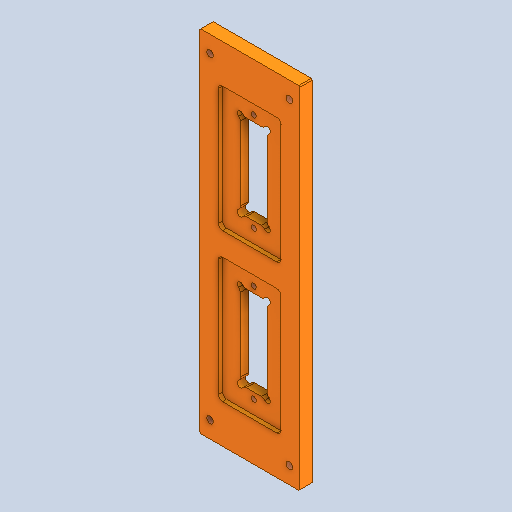
# Autodesk Inventor part: Regua DB25-berço
Saved by Autodesk Inventor 2026 (Build 300175050, 175E)
## iProperties
Created: 2025-09-19
Part Number: Regua DB25-berço
Material: Fenolite OR
Document SubType Name: Modeling
Designer: Kedson Neves
Density: 1.4 g/cm^3
Appearance: Genérico(1)
Author: Kedson Neves
Autodesk Inventor part; units mm, degrees
ref_plane "YZ Plane" through (0, 0, 0) normal (1, 0, 0) x (0, 1, 0)
ref_plane "XZ Plane" through (0, 0, 0) normal (0, 1, 0) x (-1, 0, 0)
ref_plane "XY Plane" through (0, 0, 0) normal (0, 0, 1) x (1, 0, 0)
sketch "Esboço1" plane through (0, 0, 0) normal (0, 0, 1) x (1, 0, 0)
  line L0 (24.0444, 83.9778) -> (-23.9556, 83.9778)
  line L1 (-23.9556, 83.9778) -> (-23.9556, -84.0222)
  line L2 (-23.9556, -84.0222) -> (24.0444, -84.0222)
  line L3 (24.0444, -84.0222) -> (24.0444, 83.9778)
  circle A0 centre (19.0444, 75.9778) radius 2.25
  circle A1 centre (-18.9556, 75.9778) radius 2.25
  circle A2 centre (-18.9556, -76.0222) radius 2.25
  circle A3 centre (19.0444, -76.0222) radius 2.25
  point P0 (0, 0)
  dimension "d0" = 5
  dimension "d1" = 5
  dimension "d2" = 8
  dimension "d3" = 8
  constraints: 8 end point, 4 centre point, 2 parallel, 1 horizontal, 1 perpendicular
  measures "d0" distance from line of A0.centre L3
  measures "d1" distance from line of A1.centre L1
  measures "d2" distance from line of A1.centre L0
  measures "d3" distance from line of L2 A2.centre
extrude "Extrusão1" add sketch "Esboço1" along normal blind 6
sketch "Esboço2" plane through (0, 0, 6) normal (0, 0, 1) x (1, 0, 0)
  line L0 (-10.5, 71) -> (10.5, 71)
  line L1 (10.5, 71) -> (10.5, -71)
  line L2 (10.5, -71) -> (-10.5, -71)
  line L3 (-10.5, -71) -> (-10.5, 71)
  line L4 (-10.5, 71) -> (10.5, -71) construction
  line L5 (10.5, 71) -> (-10.5, -71) construction
  line L6 (10.5, 71) -> (-10.5, 0)
  line L7 (-6.5, 56) -> (6.5, 56)
  line L8 (6.5, 56) -> (6.5, 15)
  line L9 (6.5, 15) -> (-6.5, 15)
  line L10 (-6.5, 15) -> (-6.5, 56)
  line L11 (-6.5, 56) -> (6.5, 15) construction
  line L12 (6.5, 56) -> (-6.5, 15) construction
  circle A0 centre (-6.5, 56) radius 1.5
  circle A1 centre (-6.5, 15) radius 1.5
  circle A2 centre (6.5, 15) radius 1.5
  circle A3 centre (6.5, 56) radius 1.5
  line L13 (10.5, 0) -> (-10.5, 0)
  line L14 (-6.5, -56) -> (6.5, -56)
  line L15 (6.5, -56) -> (6.5, -15)
  line L16 (6.5, -15) -> (-6.5, -15)
  line L17 (-6.5, -15) -> (-6.5, -56)
  circle A4 centre (-6.5, -56) radius 1.5
  circle A5 centre (-6.5, -15) radius 1.5
  circle A6 centre (6.5, -15) radius 1.5
  circle A7 centre (6.5, -56) radius 1.5
  point P0 (0, 0)
  point P1 (0, 35.5)
  point P2 (5, -15)
  point P3 (-5, -15)
  point P4 (-6.5, -16.5)
  point P5 (-6.5, -54.5)
  point P6 (-5, -56)
  point P7 (5, -56)
  point P8 (6.5, -54.5)
  point P9 (6.5, -16.5)
  point P10 (-5, 15)
  point P11 (5, 15)
  point P12 (6.5, 16.5)
  point P13 (6.5, 54.5)
  point P14 (5, 56)
  point P15 (-5, 56)
  point P16 (-6.5, 54.5)
  point P17 (-6.5, 16.5)
  dimension "d6" = 142
  dimension "d7" = 21
  dimension "d8" = 41
  dimension "d9" = 13
  dimension "d10" = 3
  constraints: 36 end point, 8 centre point, 8 coincident, 8 symmetric about line, 7 midpoint, 5 equal radius, 4 parallel, 3 perpendicular, 2 horizontal, 4 other
  measures "d6" distance of L0.end L1.end
  measures "d7" distance of L0.start L0.end
  measures "d8" distance of L7.end L8.end
  measures "d9" distance of L7.start L7.end
  measures "d10" diameter of A3
extrude "Extrusão2" cut sketch "Esboço2" against normal through all contours A3 L8 L7 L6 | L6 L7 A3 | A1 L10 L9 L6 | L6 L9 A1 | L7 L8 A3 L6 | L6 A3 L7 | A3 L6 A1 L10 A0 L7 | L9 L10 A1 L6 | L6 A1 L9 | A1 L6 A3 L8 A2 L9 | A0 L10 L7 | L7 L10 A0 | A2 L8 L9 | L9 L8 A2 | L17 A4 L14 | L14 A4 L17 | A4 L17 A5 L16 A6 L15 A7 L14 | A7 L15 L14 | L14 L15 A7 | A5 L16 L17 | L17 L16 A5 | A6 L16 L15 | L15 L16 A6
fillet "Arredondamento1" radius 2 16 edges at (6.5, 16.5, 3) (5, 15, 3) (-5, 15, 3) (-6.5, 16.5, 3) (-6.5, 54.5, 3) (-5, 56, 3) (5, 56, 3) (6.5, 54.5, 3) (6.5, -16.5, 3) (5, -15, 3) (-6.5, -16.5, 3) (-5, -15, 3) (-6.5, -54.5, 3) (-5, -56, 3) (5, -56, 3) (6.5, -54.5, 3)
sketch "Esboço3" plane through (0, 0, 6) normal (0, 0, 1) x (1, 0, 0)
  line L0 (6.5, 53.1277) -> (6.5, 17.8723) projected
  line L1 (6.5, 35.5) -> (-6.5, 35.5)
  line L2 (-6.5, 17.8723) -> (-6.5, 53.1277) projected
  line L3 (6.5, -53.1277) -> (6.5, -17.8723) projected
  line L4 (6.5, -35.5) -> (-6.5, -35.5)
  line L5 (-6.5, -17.8723) -> (-6.5, -53.1277) projected
  line L6 (-15, 65.5) -> (15, 65.5)
  line L7 (15, 65.5) -> (15, 5.5)
  line L8 (15, 5.5) -> (-15, 5.5)
  line L9 (-15, 5.5) -> (-15, 65.5)
  line L10 (-15, 65.5) -> (15, 5.5) construction
  line L11 (15, 65.5) -> (-15, 5.5) construction
  line L12 (-15, -5.5) -> (15, -5.5)
  line L13 (15, -5.5) -> (15, -65.5)
  line L14 (15, -65.5) -> (-15, -65.5)
  line L15 (-15, -65.5) -> (-15, -5.5)
  line L16 (-15, -5.5) -> (15, -65.5) construction
  line L17 (15, -5.5) -> (-15, -65.5) construction
  point P0 (0, 0)
  point P1 (0, 35.5)
  point P2 (0, -35.5)
  dimension "d14" = 60
  dimension "d15" = 30
  dimension "d16" = 60
  dimension "d17" = 30
  constraints: 28 end point, 10 midpoint, 4 parallel, 2 horizontal, 2 perpendicular
  measures "d14" distance of L6.end L7.end
  measures "d15" distance of L6.start L6.end
  measures "d16" distance of L12.end L13.end
  measures "d17" distance of L12.start L12.end
extrude "Extrusão3" cut sketch "Esboço3" against normal blind 2
fillet "Arredondamento2" radius 2 8 edges at (15, 65.5, 5) (-15, 65.5, 5) (-15, 5.5, 5) (15, 5.5, 5) (15, -5.5, 5) (-15, -5.5, 5) (-15, -65.5, 5) (15, -65.5, 5)
sketch "Esboço4" plane through (0, 0, 4) normal (0, 0, 1) x (1, 0, 0)
  line L0 (6.5, 17.8723) -> (6.5, 53.1277) projected
  line L1 (6.5, 35.5) -> (-6.5, 35.5)
  line L2 (-6.5, 53.1277) -> (-6.5, 17.8723) projected
  line L3 (6.5, -53.1277) -> (6.5, -17.8723) projected
  line L4 (6.5, -35.5) -> (-6.5, -35.5)
  line L5 (-6.5, -17.8723) -> (-6.5, -53.1277) projected
  point P0 (0, 0)
  point P1 (0, 12)
  point P2 (0, 59)
  point P3 (0, -12)
  point P4 (0, -59)
  dimension "d21" = 23.5
  dimension "d22" = 23.5
  dimension "d23" = 6.5
  dimension "d24" = 6.5
  dimension "d25" = 23.5
  dimension "d26" = 23.5
  dimension "d27" = 6.5
  dimension "d28" = 6.5
  constraints: 4 end point, 4 midpoint
  measures "d21" distance from line of L1 point (0, 59)
  measures "d22" distance from line of L1 point (0, 12)
  measures "d23" distance from line of L2 point (0, 12)
  measures "d24" distance from line of L2 point (0, 59)
  measures "d25" distance from line of L4 point (0, -12)
  measures "d26" distance from line of point (0, -59) L4
  measures "d27" distance from line of L5 point (0, -12)
  measures "d28" distance from line of L5 point (0, -59)
hole "Furo1" at (0, 12, 4) at (0, 59, 4) at (0, -12, 4) at (0, -59, 4) direction (0, 0, -1) diameter 2.459 depth 4 thread size "M3x0.5" class "6H" standard "ISO Metric profile"
offset faces "Tamanho1" outward 1 faces at (16.8235, 76.3387, 2) (-21.1765, 76.3387, 2) (-16.7348, -76.3831, 4) (16.8235, -75.6613, 2)
sketch "Esboço5" plane through (0, 0, 6) normal (0, 0, 1) x (1, 0, 0)
  circle A0 centre (19.0444, 75.9778) radius 1.25 projected
  circle A1 centre (-18.9556, 75.9778) radius 1.25 projected
  circle A2 centre (-18.9556, -76.0222) radius 1.25 projected
  circle A3 centre (19.0444, -76.0222) radius 1.25 projected
  point P0 (0, 0)
  constraints: 4 coincident
hole "Furo2" at (19.0444, 75.9778, 6) at (-18.9556, 75.9778, 6) at (-18.9556, -76.0222, 6) at (19.0444, -76.0222, 6) direction (0, 0, -1) diameter 3.242 depth 6 thread size "M4x0.7" class "6H" standard "ISO Metric profile"
chamfer "Chanfro1" distance 0.5 angle 45 4 edges at (24.0444, 83.9778, 3) (-23.9556, 83.9778, 3) (24.0444, -84.0222, 3) (-23.9556, -84.0222, 3)
